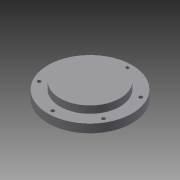
# Autodesk Inventor part: bat_endcap
Saved by Autodesk Inventor 2015 (Build 190159000, 159)
## iProperties
Created: 2015-09-14
Part Number: bat_endcap
Material: Generic
Document SubType Name: Modeling
Designer: Thomas
Density: 1 g/cm^3
Appearance: Default
Author: Thomas
Autodesk Inventor part; units mm, degrees
ref_plane "YZ Plane" through (0, 0, 0) normal (1, 0, 0) x (0, 1, 0)
ref_plane "XZ Plane" through (0, 0, 0) normal (0, 1, 0) x (-1, 0, 0)
ref_plane "XY Plane" through (0, 0, 0) normal (0, 0, 1) x (1, 0, 0)
sketch "Sketch1" plane through (0, 0, 0) normal (0, 1, 0) x (-1, 0, 0)
  circle A0 centre (0, 0) radius 35
  circle A1 centre (0, 0) radius 25
  dimension "d1" = 70
  dimension "d2" = 50
  constraints: 2 centre point, 2 coincident
  measures "d1" diameter of A0
  measures "d2" diameter of A1
sketch "Sketch2" plane through (0, 0, 0) normal (0, 1, 0) x (-1, 0, 0)
  circle A0 centre (0, 0) radius 25
  circle A1 centre (0, 0) radius 35
  dimension "d3" = 50
  dimension "d4" = 70
  constraints: 2 centre point, 2 coincident
  measures "d3" diameter of A0
  measures "d4" diameter of A1
extrude "Extrusion1" add sketch "Sketch1" along normal blind 7
extrude "Extrusion2" add sketch "Sketch2" along normal blind 13 contours A0
sketch "Sketch3" plane through (0, 0, 0) normal (0, -1, 0) x (1, 0, 0)
  line L0 (0, 0) -> (0, -35)
  circle A0 centre (0, 0) radius 35 projected
  line L1 (0, 35) -> (0, 0)
  line L2 (30.3109, -17.5) -> (0, -35)
  line L3 (0, -35) -> (-30.3109, -17.5)
  line L4 (-30.3109, -17.5) -> (-30.3109, 17.5)
  line L5 (-30.3109, 17.5) -> (0, 35)
  line L6 (0, 35) -> (30.3109, 17.5)
  line L7 (30.3109, 17.5) -> (30.3109, -17.5)
  line L8 (0, 0) -> (30.3109, 17.5)
  line L9 (0, 0) -> (0, 35)
  line L10 (0, 0) -> (-30.3109, 17.5)
  line L11 (0, 0) -> (-30.3109, -17.5)
  line L12 (0, 0) -> (0, -35)
  line L13 (0, 0) -> (30.3109, -17.5)
  line L14 (30.3109, 17.5) -> (26.8468, 15.5)
  line L15 (26.8468, 15.5) -> (26.8468, -15.5)
  line L16 (0, -35) -> (0, -31)
  line L17 (-30.3109, -17.5) -> (-26.8468, -15.5)
  line L18 (0, 35) -> (0, 31)
  line L19 (-30.3109, 17.5) -> (-26.8468, 15.5)
  dimension "d9" = 4
  dimension "d10" = 4
  dimension "d11" = 4
  dimension "d12" = 4
  dimension "d13" = 4
  constraints: 40 end point, 7 point on line, 5 collinear, 3 point on circle, 1 coincident, 1 parallel, 1 vertical, 13 other
  measures "d9" distance of L6.end L14.end
  measures "d10" distance of L2.end L16.end
  measures "d11" distance of L3.end L17.end
  measures "d12" distance of L5.end L18.end
  measures "d13" distance of L4.end L19.end
hole "Hole1" at (26.8468, 0, 15.5) at (26.8468, 0, -15.5) at (0, 0, -31) at (-26.8468, 0, -15.5) at (-26.8468, 0, 15.5) at (0, 0, 31) direction (0, 1, 0) diameter 3 end through all
body "Solid1"
